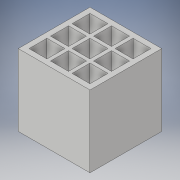
# Autodesk Inventor part: Gold
Saved by Autodesk Inventor 2019 (Build 230136000, 136)
## iProperties
Created: 2018-10-25
Part Number: Gold
Material: Generic
Document SubType Name: Modeling
Designer: User
Density: 1 g/cm^3
Appearance: Default
Author: User
Autodesk Inventor part; units mm, degrees
ref_plane "YZ Plane" through (0, 0, 0) normal (1, 0, 0) x (0, 1, 0)
ref_plane "XZ Plane" through (0, 0, 0) normal (0, 1, 0) x (-1, 0, 0)
ref_plane "XY Plane" through (0, 0, 0) normal (0, 0, 1) x (1, 0, 0)
sketch "Sketch1" plane through (0, 0, 0) normal (0, 0, 1) x (1, 0, 0)
  line L0 (0, 0) -> (50.8, 0)
  line L1 (50.8, 0) -> (50.8, 50.8)
  line L2 (50.8, 50.8) -> (0, 50.8)
  line L3 (0, 50.8) -> (0, 0)
  dimension "d0" = 50.8
  dimension "d1" = 50.8
  constraints: 8 end point, 2 parallel, 1 horizontal, 1 perpendicular
  measures "d0" distance of L2.end L1.end
  measures "d1" distance of L1.end L0.end
extrude "Extrusion1" add sketch "Sketch1" along normal blind 50.8
sketch "Sketch2" plane through (0, 50.8, 0) normal (0, 1, 0) x (1, 0, 0)
  line L0 (50.8, 0) -> (0, 0) projected
  line L1 (0, 0) -> (0, -50.8) projected
  line L2 (50.8, -50.8) -> (0, -50.8) projected
  line L3 (50.8, 0) -> (50.8, -50.8) projected
  line L4 (46.99, -46.99) -> (34.29, -46.99)
  line L5 (34.29, -46.99) -> (34.29, -34.29)
  line L6 (34.29, -34.29) -> (46.99, -34.29)
  line L7 (46.99, -34.29) -> (46.99, -46.99)
  line L8 (19.05, -46.99) -> (19.05, -34.29)
  line L9 (19.05, -34.29) -> (31.75, -34.29)
  line L10 (31.75, -34.29) -> (31.75, -46.99)
  line L11 (31.75, -46.99) -> (19.05, -46.99)
  line L12 (3.81, -46.99) -> (3.81, -34.29)
  line L13 (3.81, -34.29) -> (16.51, -34.29)
  line L14 (16.51, -34.29) -> (16.51, -46.99)
  line L15 (16.51, -46.99) -> (3.81, -46.99)
  line L16 (34.29, -31.75) -> (34.29, -19.05)
  line L17 (34.29, -19.05) -> (46.99, -19.05)
  line L18 (46.99, -19.05) -> (46.99, -31.75)
  line L19 (46.99, -31.75) -> (34.29, -31.75)
  line L20 (19.05, -31.75) -> (19.05, -19.05)
  line L21 (19.05, -19.05) -> (31.75, -19.05)
  line L22 (31.75, -19.05) -> (31.75, -31.75)
  line L23 (31.75, -31.75) -> (19.05, -31.75)
  line L24 (3.81, -31.75) -> (3.81, -19.05)
  line L25 (3.81, -19.05) -> (16.51, -19.05)
  line L26 (16.51, -19.05) -> (16.51, -31.75)
  line L27 (16.51, -31.75) -> (3.81, -31.75)
  line L28 (34.29, -16.51) -> (34.29, -3.81)
  line L29 (34.29, -3.81) -> (46.99, -3.81)
  line L30 (46.99, -3.81) -> (46.99, -16.51)
  line L31 (46.99, -16.51) -> (34.29, -16.51)
  line L32 (19.05, -16.51) -> (19.05, -3.81)
  line L33 (19.05, -3.81) -> (31.75, -3.81)
  line L34 (31.75, -3.81) -> (31.75, -16.51)
  line L35 (31.75, -16.51) -> (19.05, -16.51)
  line L36 (3.81, -16.51) -> (3.81, -3.81)
  line L37 (3.81, -3.81) -> (16.51, -3.81)
  line L38 (16.51, -3.81) -> (16.51, -16.51)
  line L39 (16.51, -16.51) -> (3.81, -16.51)
  dimension "d4" = 12.7
  dimension "d5" = 12.7
  dimension "d6" = 3.81
  dimension "d7" = 3.81
  dimension "d10" = 15.24
  dimension "d13" = 15.24
  constraints: 72 end point, 2 horizontal, 2 parallel, 1 perpendicular, 1 vertical, 64 other
  measures "d4" distance of L5.end L6.end
  measures "d5" distance of L4.end L5.end
  measures "d6" distance between parallel lines of L2 L4
  measures "d7" distance between parallel lines of L3 L7
  measures "d10" distance of L4.end L8.start
  measures "d13" distance of L4.end L16.start
extrude "Extrusion2" cut sketch "Sketch2" against normal through all contours L4 L5 L6 L7 | L8 L9 L10 L11 | L12 L13 L14 L15 | L16 L17 L18 L19 | L20 L21 L22 L23 | L24 L25 L26 L27 | L28 L29 L30 L31 | L32 L33 L34 L35 | L36 L37 L38 L39
body "Solid1"
